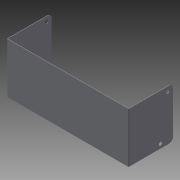
# Autodesk Inventor part: radio_base
Saved by Autodesk Inventor 2014 (Build 180170000, 170)
## iProperties
Created: 2014-04-06
Part Number: radio_base
Material: Generic
Document SubType Name: Sheet Metal
Designer: Tyler
Density: 1 g/cm^3
Sheet Metal Rule: Default_mm
Appearance: Default
Author: Tyler
Autodesk Inventor part; units mm, degrees
ref_plane "YZ Plane" through (0, 0, 0) normal (1, 0, 0) x (0, 1, 0)
ref_plane "XZ Plane" through (0, 0, 0) normal (0, 1, 0) x (-1, 0, 0)
ref_plane "XY Plane" through (0, 0, 0) normal (0, 0, 1) x (1, 0, 0)
sketch "Sketch1" plane through (0, 0, 0) normal (0, 1, 0) x (-1, 0, 0)
  line L0 (-72, 30) -> (72, 30)
  line L1 (72, 30) -> (72, -30)
  line L2 (72, -30) -> (-72, -30)
  line L3 (-72, -30) -> (-72, 30)
  point P0 (0, 0)
  dimension "d0" = 144
  dimension "d1" = 60
  dimension "d2" = 72
  dimension "d3" = 30
  measures "d0" distance of L0.start L0.end
  measures "d1" distance of L0.end L1.end
  measures "d2" distance from line of point (0, 0) L1
  measures "d3" distance from line of L0 point (0, 0)
extrude "Plate1" add sketch "Sketch1" along normal blind 0.5
sketch "Sketch3" plane through (72, 0.5, -30) normal (1, 0, 0) x (0, 1, 0)
  line L0 (0, 60) -> (0, 0)
  line L1 (0, 0) -> (52.5, 0)
  line L2 (52.5, 0) -> (52.5, 60)
  line L3 (52.5, 60) -> (0, 60)
  constraints: 6 end point, 1 horizontal, 1 perpendicular, 1 vertical
edge flange "Flange1" height 53 angle 90 thickness 0.5 bend radius 0.5 thickness toward (1, 0, 0) relief tear relief width 0.5 relief depth 0.25 corner gap 0.5 corner form 0 edges at (72, 0.5, 0) (-72, 0.5, 0) wall of the first edge with corners at (72, 0.5, 30) (72, 0.5, -30) (72, 53, -30) (72, 53, 30)
bend "Bend1"
corner "Corner1"
fillet "Corner Round1" radius 5 4 edges at (-72.25, 53, -30) (-72.25, 53, 30) (72.25, 53, -30) (72.25, 53, 30)
sketch "Sketch4" plane through (72.5, 1, 30) normal (1, 0, 0) x (0, 0, -1)
  line L0 (5, 52) -> (55, 52) projected
  line L1 (60, 47) -> (60, 0) projected
  line L2 (5.7596, 45.6824) -> (55, 37) construction
  point P0 (30, -1)
  dimension "d19" = 5
  dimension "d20" = 15
  dimension "d21" = 50
  dimension "d22" = 10
  constraints: 2 end point
  measures "d19" distance from line of L1 L2.end
  measures "d20" distance from line of L0 L2.end
  measures "d21" distance of L2.start L2.end
  measures "d22" angle of L0 L2
hole "Hole1" at (72.5, 38, -25) at (72.5, 46.6824, 24.2404) direction (-1, 0, 0) diameter 4 end through all
equation "\"d28\" = Thickness"
equation "\"d8\" = BendReliefWidth"
equation "\"d9\" = BendReliefDepth"
equation "\"d10\" = MinimumRemnant"
equation "\"d11\" = BendRadius"
equation "\"d14\" = BendRadius"
equation "\"d15\" = CornerReliefSize"
equation "\"d16\" = GapSize"
equation "\"d17\" = JacobiRadiusSize"
equation "\"d2\" = 0.5 * d0"
equation "\"d3\" = 0.5 * d1"
equation "\"BendRadius\" = Thickness"
equation "\"BendReliefWidth\" = Thickness"
equation "\"BendReliefDepth\" = 0.5 * Thickness"
equation "\"CornerReliefSize\" = 4 * Thickness"
equation "\"MinimumRemnant\" = 2 * Thickness"
equation "\"TransitionRadius\" = BendRadius"
equation "\"JacobiRadiusSize\" = BendRadius"
equation "\"GapSize\" = Thickness"
equation "\"d4\" = BendRadius"
equation "\"Thickness\" = 0.5"
body "Solid1"
